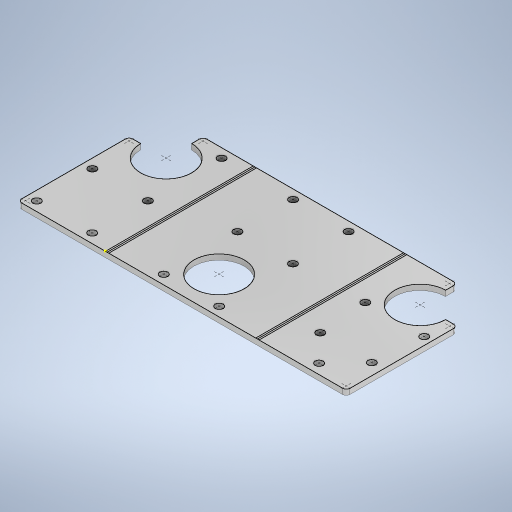
# Autodesk Inventor part: axis_3_top_frame
Saved by Autodesk Inventor 2024.2 (Build 282272000, 272)
## iProperties
Created: 2023-12-26
Part Number: axis_3_top_frame
Material: Aluminum 6061-AHC
Document SubType Name: Modeling
Designer: chanh
Density: 2.7 g/cm^3
Appearance: Aluminum - Dark
Author: chanh
Autodesk Inventor part; units mm, degrees
ref_plane "YZ Plane" through (0, 0, 0) normal (1, 0, 0) x (0, 1, 0)
ref_plane "XZ Plane" through (0, 0, 0) normal (0, 1, 0) x (-1, 0, 0)
ref_plane "XY Plane" through (0, 0, 0) normal (0, 0, 1) x (1, 0, 0)
sketch "Sketch1" plane through (0, 0, 0) normal (0, 1, 0) x (-1, 0, 0)
  line L0 (-0.4496, -40.1) -> (-0.4496, 0)
  line L1 (-41.2289, 0) -> (-41.2289, -40.1)
  circle A0 centre (6.095, -37.6) radius 1.05
  circle A1 centre (21.145, -17.6) radius 1.05
  circle A2 centre (6.095, -17.6) radius 1.05
  circle A3 centre (21.145, -2.5) radius 1.05
  circle A4 centre (6.095, -2.5) radius 1.05
  circle A5 centre (-28.3643, -37.6) radius 1.05
  circle A6 centre (-13.3143, -37.6) radius 1.05
  circle A7 centre (-28.3643, -22.5) radius 1.05
  circle A8 centre (-13.3143, -22.5) radius 1.05
  circle A9 centre (-28.3643, -2.5) radius 1.05
  circle A10 centre (-13.3143, -2.5) radius 1.05
  circle A11 centre (-20.8393, -10) radius 6.8
  circle A12 centre (-47.2986, -23.2) radius 1.05
  circle A13 centre (-63.2986, -23.2) radius 1.05
  circle A14 centre (-48.2986, -9.98) radius 1.05
  circle A15 centre (-62.2986, -9.98) radius 1.05
  circle A16 centre (-55.2986, -2.68) radius 1.05
  arc A17 (23.69, -1) -> (22.69, 0) centre (22.69, -1) ccw
  arc A18 (-64.3686, 0) -> (-65.3686, -1) centre (-64.3686, -1) ccw
  line L2 (-65.3686, -29.1) -> (-65.3686, -1)
  arc A19 (-65.3686, -29.1) -> (-64.3686, -30.1) centre (-64.3686, -29.1) ccw
  line L3 (-64.3686, -30.1) -> (-62.1986, -30.1)
  arc A20 (-55.2986, -39.1) -> (-54.2986, -40.1) centre (-54.2986, -39.1) ccw
  line L4 (-55.2986, -37) -> (-55.2986, -39.1)
  arc A21 (22.69, -30.1) -> (23.69, -29.1) centre (22.69, -29.1) ccw
  line L5 (20.52, -30.1) -> (22.69, -30.1)
  arc A22 (12.62, -40.1) -> (13.62, -39.1) centre (12.62, -39.1) ccw
  line L6 (13.62, -39.1) -> (13.62, -37)
  arc A23 (20.52, -30.1) -> (13.62, -37) centre (13.62, -30.1) ccw
  arc A24 (-55.2986, -37) -> (-62.1986, -30.1) centre (-55.2986, -30.1) ccw
  line L7 (23.69, -1) -> (23.69, -29.1)
  line L8 (-64.3686, 0) -> (22.69, 0)
  line L9 (12.62, -40.1) -> (-54.2986, -40.1)
  line L10 (-41.6786, -40.1) -> (-41.6786, 0)
  line L11 (-40.7793, 0) -> (-40.7793, -40.1)
  line L12 (-0.8993, -40.1) -> (-0.8993, 0)
  line L13 (0, 0) -> (0, -40.1)
  point P0 (0, 0)
  constraints: 28 end point, 25 centre point, 16 point on circle, 12 point on line, 10 vertical, 4 horizontal, 79 other
extrude "Extrusion1" add sketch "Sketch1" against normal blind 1.5
body "Solid1"
